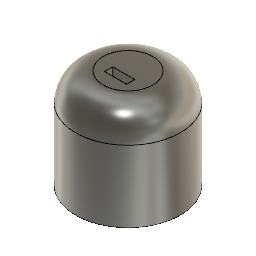
3D printed cover (Autodesk Fusion 360 design; units mm, degrees)
Autodesk Fusion 360 part; units mm, degrees
sketch "bottom sketch" plane through (0, 0, 0) normal (0, 0, 1) x (1, 0, 0)
  line L0 (0, 0) -> (11.5, 0)
  line L1 (-11.4997, -1.5051) -> (-11.5005, 2.4949)
  arc A0 (-11.4011, -1.5051) -> (11.4018, -1.5) centre (0, 0) ccw
  arc A1 (11.2261, 2.4949) -> (-11.2287, 2.4831) centre (0, 0) ccw
  line L2 (-11.5001, 0.4949) -> (-19.0001, 0.4932)
  line L3 (11.5, 0) -> (19, 0)
  circle A2 centre (0, 0) radius 19
  line L4 (11.4997, 1.5) -> (11.5003, -1.5)
  line L5 (0, 0) -> (5.9167, 136.7817)
  line L6 (-11.5005, 2.4949) -> (11.5003, 2.4949)
  line L7 (11.5003, 2.4949) -> (11.5003, -1.5)
  line L8 (11.5003, -1.5) -> (-11.5005, -1.5)
  line L9 (-11.5005, -1.5) -> (-11.5005, 2.4949)
  dimension "d3" = 23
  dimension "d4" = 1.5
  dimension "d5" = 1.5
  dimension "d6" = 23
  dimension "d7" = 4
  dimension "d10" = 7.5
  dimension "d11" = 7.5
  constraint coincident L0.start A0.centre
  constraint horizontal L0
  constraint concentric A0 A1
  constraint midpoint L1 L2.start
  constraint perpendicular L1 L2
  constraint coincident L3.end A2
  constraint horizontal L6
  constraint vertical L7
  constraint horizontal L8
  constraint vertical L9
  constraint coincident L6 A1.start
  measures "d3" diameter of A0
  measures "d4" distance of L0.end L4.start
  measures "d5" distance of L0.end L4.end
  measures "d6" distance of L4.end L1.start
  measures "d7" distance of L1.start L1.end
  measures "d10" distance of L2.start L2.end
  measures "d11" distance of L0.end L3.end
extrude "Extrude1" add sketch "bottom sketch" along normal blind 21
sketch "Sketch2" plane through (0, 0, 21) normal (0, 0, 1) x (-1, 0, 0)
  circle A0 centre (0, 0) radius 19
  line L0 (0, 0) -> (-6, -0.0013)
  line L1 (-6, -0.0013) -> (6, -0.0013)
  line L2 (6, -0.0013) -> (6, 6.9987)
  line L3 (6, 6.9987) -> (-6, 6.9987)
  line L4 (-6, 6.9987) -> (-6, -0.0013)
  dimension "d15" = 6
  dimension "d16" = 12
  dimension "d17" = 7
  constraint coincident A0.centre L0.start
  constraint horizontal L1
  constraint vertical L2
  constraint horizontal L3
  constraint vertical L4
  measures "d15" distance of A0.centre L0.end
  measures "d16" distance of L0.end L1.end
  measures "d17" distance of L0.end L3.end
extrude "Extrude2" add sketch "Sketch2" along normal blind 5
sketch "Sketch8" plane through (0, 0, 0) normal (0, 0, 1) x (1, 0, 0)
extrude "Extrude3" cut 1 faces at (0, -4.6658, 21) along direction (0, 0, -1) blind 30
sketch "Sketch6" plane through (0, 0, 26) normal (0, 0, 1) x (-1, 0, 0)
  line L0 (6, 6.9987) -> (6, -0.0013)
  line L1 (-6, -0.0013) -> (-6, 6.9987)
  line L2 (-6, 6.9987) -> (6, 6.9987)
  circle A0 centre (0, 0) radius 19
  line L3 (-11.4997, -1.5) -> (11.4997, -1.5)
  line L4 (11.4997, -1.5) -> (11.4997, 1.5051)
  line L5 (11.4997, 1.5051) -> (-11.4997, 1.5051)
  line L6 (-11.4997, 1.5051) -> (-11.4997, -1.5)
  line L7 (6, -0.0013) -> (-6, -0.0013)
  constraint horizontal L3
  constraint vertical L4
  constraint horizontal L5
  constraint vertical L6
extrude "Extrude4" add sketch "Sketch6" along normal blind 5 contours L0 L1 L3 L4 L5 L6 L7 | L0 L1 L5 L7 | A0
sketch "Sketch7" plane through (0, 0, 31) normal (0, 0, 1) x (-1, 0, 0)
  line L0 (-6, 6.9987) -> (6, 6.9987)
  line L1 (6, 6.9987) -> (6, 1.5051)
  line L2 (6, 1.5051) -> (-6, 1.5051)
  line L3 (-6, 1.5051) -> (-6, 6.9987)
  circle A0 centre (0, 0) radius 19
  line L4 (-4, 1.5) -> (-4, 7)
  line L5 (-4, 1.5) -> (4, 1.5)
  line L6 (4, 1.5) -> (4, 4.5)
  line L7 (4, 4.5) -> (-4, 4.5)
  line L8 (-4, 4.5) -> (-4, 1.5)
  dimension "d28" = 8
  dimension "d29" = 3
  constraint vertical L4
  constraint horizontal L5
  constraint vertical L6
  constraint horizontal L7
  constraint vertical L8
  measures "d28" distance of L4.start L5.end
  measures "d29" distance of L4.start L7.end
extrude "Extrude5" add sketch "Sketch7" along normal blind 5 contours L0 L2 L3 L4 L8 | L0 L1 L2 L4 L6 L7 | A0
fillet "Fillet1" radius 10 1 edges at (17.7142, 6.8707, 36)
extrude "Extrude6" cut sketch "bottom sketch" along normal blind 26 contours L0 L4 L5 L6 L7 | L0 L1 L4 L5 L6 L7 L8 L9
sketch "Sketch9" plane through (0, 0, 0) normal (0, 0, -1) x (1, 0, 0)
  line L0 (-11.4997, 1.5) -> (-6, 1.5)
  line L1 (-6, 1.5) -> (-6, 6.9987)
  line L2 (-6, 6.9987) -> (6, 6.9987)
  line L3 (6, 6.9987) -> (6, 1.5)
  line L4 (6, 1.5) -> (11.5003, 1.5)
  line L5 (11.5003, 1.5) -> (11.5, 0)
  line L6 (11.5, 0) -> (11.5003, 0)
  line L7 (11.5003, 0) -> (11.5003, -2.4949)
  line L8 (-11.5005, -2.4949) -> (-11.4997, 1.5)
  circle A0 centre (0, 0) radius 19
  line L9 (-6, 1.5) -> (-11.5, 1.5)
  line L10 (-11.5, 1.5) -> (-11.5, 3.5)
  line L11 (-11.5, 3.5) -> (-6, 3.5)
  line L12 (-6, 3.5) -> (-6, 1.5)
  line L13 (6, 1.5) -> (11.5, 1.5)
  line L14 (11.5, 1.5) -> (11.5, 3.5)
  line L15 (11.5, 3.5) -> (6, 3.5)
  line L16 (6, 3.5) -> (6, 1.5)
  line L17 (-11.4997, -2.4949) -> (-11.4997, -2.1949)
  line L18 (11.5003, -2.1949) -> (11.5003, -2.4949)
  line L19 (11.5003, -2.4949) -> (-11.4997, -2.4949)
  line L20 (-11.4997, -2.4949) -> (-11.4997, -2.6949)
  line L21 (-11.4997, -2.6949) -> (11.5003, -2.6949)
  line L22 (11.5003, -2.6949) -> (11.5003, -2.4949)
  dimension "d35" = 5.5
  dimension "d36" = 2
  dimension "d37" = 5.5
  dimension "d38" = 2
  dimension "d39" = 23
  dimension "d40" = 0.3
  dimension "d41" = 23
  dimension "d42" = 0.2
  constraint horizontal L9
  constraint vertical L10
  constraint horizontal L11
  constraint vertical L12
  constraint coincident L0.end L1.start
  constraint horizontal L13
  constraint vertical L14
  constraint horizontal L15
  constraint vertical L16
  constraint coincident L3.end L4.start
  constraint vertical L17
  constraint vertical L18
  constraint coincident L7.end L18.end
  constraint horizontal L19
  constraint vertical L20
  constraint horizontal L21
  constraint vertical L22
  measures "d35" distance of L0.end L9.end
  measures "d36" distance of L0.end L11.end
  measures "d37" distance of L3.end L13.end
  measures "d38" distance of L3.end L15.end
  measures "d39" distance of L7.end L17.start
  measures "d40" distance of L7.end L18.start
  measures "d41" distance of L7.end L17.start
  measures "d42" distance of L7.end L21.end
extrude "Extrude7" cut sketch "Sketch9" against normal blind 26 contours L0 L1 L9 L10 L11 L12 | L3 L4 L13 L14 L15 L16
equation "thickness = 4 mm"
equation "innerdiameter = 23 mm"
equation "d7 = thickness"
equation "wallthickness = 7.5 mm"
equation "d10 = wallthickness"
equation "d11 = wallthickness"
